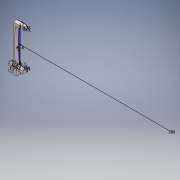
# Autodesk Inventor part: RightClip
Saved by Autodesk Inventor 2017 (Build 210142000, 142)
## iProperties
Created: 2017-12-02
Part Number: RightClip
Material: Generic
Document SubType Name: Modeling
Designer: Max
Density: 1 g/cm^3
Appearance: Default
Author: Max
Autodesk Inventor part; units mm, degrees
ref_plane "YZ Plane" through (0, 0, 0) normal (1, 0, 0) x (0, 1, 0)
ref_plane "XZ Plane" through (0, 0, 0) normal (0, 1, 0) x (-1, 0, 0)
ref_plane "XY Plane" through (0, 0, 0) normal (0, 0, 1) x (1, 0, 0)
sketch "Sketch1" plane through (0, 0, 0) normal (0, 1, 0) x (-1, 0, 0)
  line L0 (10.2, -3) -> (10.2, -49.6)
  line L1 (10.2, -49.6) -> (0.5, -49.6)
  line L2 (0.5, -49.6) -> (0.5, -48.85)
  line L3 (0.5, -48.85) -> (0, -48.85)
  line L4 (0, -48.85) -> (0, -49.6)
  line L5 (0.5, -3) -> (0.5, -3.75)
  line L6 (0.5, -3.75) -> (0, -3.75)
  line L7 (0, -3.75) -> (0, -3)
  line L8 (0, -3) -> (0, 0)
  line L9 (0, 0) -> (13.2, 0)
  line L10 (13.2, 0) -> (13.2, -50.35)
  line L11 (13.2, -52.6) -> (12.7, -52.6)
  line L12 (0, -52.6) -> (0, -49.6)
  line L13 (10.2, -3) -> (0.5, -3)
  line L14 (8.7, -59.3) -> (19.7, -59.3)
  line L15 (19.7, -59.3) -> (19.7, -57.6)
  line L16 (19.7, -57.6) -> (12.7, -57.6)
  line L17 (12.7, -57.6) -> (12.7, -52.6)
  line L18 (12.7, -52.6) -> (13.2, -52.6)
  line L19 (19.7, -52.6) -> (19.7, -50.35)
  line L20 (19.7, -50.35) -> (13.2, -50.35)
  line L21 (8.7, -59.3) -> (8.7, -52.6)
  arc A0 (10.2, -49.6) -> (10.2, -3) centre (-188.4381, -26.3) ccw
  line L22 (12.7, -52.6) -> (12.7, -52.6)
  line L23 (13.2, -52.6) -> (19.7, -52.6)
  line L24 (13.2, -52.6) -> (13.2, -52.6)
  line L25 (8.7, -52.6) -> (0, -52.6)
  point P0 (0, 0)
  dimension "d1" = 9.7
  dimension "d2" = 0.75
  dimension "d3" = 0.5
  dimension "d6" = 0.5
  dimension "d10" = 46.6
  dimension "d11" = 3
  dimension "d13" = 0.75
  dimension "d14" = 3
  dimension "d15" = 3
  dimension "d16" = 5
  dimension "d19" = 7
  dimension "d23" = 4.5
  dimension "d25" = 200
  dimension "d30" = 2.25
  dimension "d31" = 2.25
  dimension "d32" = 1.7
  dimension "d33" = 4
  constraints: 52 end point, 28 perpendicular, 6 point on line, 2 horizontal, 2 point on circle, 1 centre point, 1 coincident, 1 parallel
  measures "d1" distance of L0.end L1.end
  measures "d2" distance of L1.end L2.end
  measures "d3" distance of L2.end L3.end
  measures "d6" distance of L5.end L6.end
  measures "d10" distance of L0.start L0.end
  measures "d11" distance between parallel lines of L10 L0
  measures "d13" distance between parallel lines of L6 L13
  measures "d14" distance between parallel lines of L9 L13
  measures "d15" distance between parallel lines of L11 L1
  measures "d16" distance of L16.end L18.start
  measures "d19" distance of L18.start L19.start
  measures "d23" distance between parallel lines of L10 L21
  measures "d25" radius of A0
  measures "d30" distance from line of L11 L10.end
  measures "d31" distance of L19.start L19.end
  measures "d32" distance of L14.end L15.end
  measures "d33" distance between parallel lines of L21 L17
extrude "Extrusion2" add sketch "Sketch1" against normal blind 5 contours L13 L5 L6 L7 L8 L9 L10 L20 L19 L23 L11 L17 L16 L15 L14 L21 L25 L12 L4 L3 L2 L1 A0
body "Solid1"
